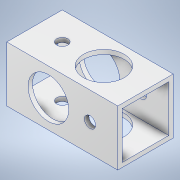
# Autodesk Inventor part: ロボットベース15x15x30
Saved by Autodesk Inventor 2020.3 (Build 243373000, 373)
## iProperties
Created: 2020-07-04
Part Number: ロボットベース15x15x30
Material: アルミニウム 6061
Document SubType Name: Modeling
Designer: totot
Density: 2.7 g/cm^3
Appearance: アルミニウム - フラット
Mass: 4.65802 g
Surface Area: 31.3598 cm^2
Volume: 1.72519 cm^3
Author: totot
Autodesk Inventor part; units mm, degrees
ref_plane "YZ Plane" through (0, 0, 0) normal (1, 0, 0) x (0, 1, 0)
ref_plane "XZ Plane" through (0, 0, 0) normal (0, 1, 0) x (-1, 0, 0)
ref_plane "XY Plane" through (0, 0, 0) normal (0, 0, 1) x (1, 0, 0)
sketch "スケッチ1" plane through (0, 0, 0) normal (1, 0, 0) x (0, 1, 0)
  line L0 (0, 0) -> (-15, 0)
  line L1 (-15, 0) -> (-15, 15)
  line L2 (-15, 15) -> (0, 15)
  line L3 (0, 15) -> (0, 0)
  line L4 (-13.8, 1.2) -> (-1.2, 1.2)
  line L5 (-1.2, 1.2) -> (-1.2, 13.8)
  line L6 (-1.2, 13.8) -> (-13.8, 13.8)
  line L7 (-13.8, 13.8) -> (-13.8, 1.2)
  dimension "d0" = 15
  dimension "d1" = 15
  dimension "d2" = 1.2
  dimension "d3" = 1.2
  dimension "d4" = 1.2
  dimension "d5" = 1.2
  constraints: 16 end point, 4 parallel, 2 horizontal, 2 perpendicular
  measures "d0" distance of L1.end L2.end
  measures "d1" distance of L0.end L1.end
  measures "d2" distance between parallel lines of L7 L1
  measures "d3" distance between parallel lines of L4 L0
  measures "d4" distance between parallel lines of L3 L5
  measures "d5" distance between parallel lines of L2 L6
extrude "押し出し1" add sketch "スケッチ1" along normal blind 30
sketch "スケッチ2" plane through (0, -15, 15) normal (0, 0, 1) x (1, 0, 0)
  line L0 (0, 0) -> (30, 0) projected
  line L1 (30, 15) -> (30, 0) projected
  point P0 (0, 15)
  point P1 (22.5, 7.5)
  dimension "d8" = 7.5
  dimension "d9" = 7.5
  measures "d8" distance from line of point (22.5, 7.5) L0
  measures "d9" distance from line of point (22.5, 7.5) L1
sketch "スケッチ3" plane through (0, 0, 15) normal (0, 1, 0) x (1, 0, 0)
  line L0 (0, 15) -> (0, 0) projected
  line L1 (0, 15) -> (30, 15) projected
  point P0 (7.5, 7.5)
  dimension "d10" = 7.5
  dimension "d11" = 7.5
  measures "d10" distance from line of point (7.5, 7.5) L0
  measures "d11" distance from line of point (7.5, 7.5) L1
hole "穴1" at (22.5, -7.5, 15) direction (0, 0, -1) diameter 3 end through all
hole "穴2" at (7.5, 0, 7.5) direction (0, -1, 0) diameter 3 end through all
sketch "スケッチ4" plane through (0, -15, 15) normal (0, 0, 1) x (1, 0, 0)
  circle A0 centre (22.5, 7.5) radius 1.5 projected
  line L0 (0, 15) -> (0, 0) projected
  line L1 (0, 15) -> (30, 15) projected
  point P0 (11.25, 7.5)
  dimension "d26" = 22.5
  dimension "d27" = 11.25
  dimension "d28" = 7.5
  measures "d26" distance from line of A0.centre L0
  measures "d27" distance from line of point (11.25, 7.5) L0
  measures "d28" distance from line of L1 point (11.25, 7.5)
hole "穴3" at (11.25, -7.5, 15) direction (0, 0, -1) diameter 11 end through all
sketch "スケッチ5" plane through (0, 0, 15) normal (0, 1, 0) x (1, 0, 0)
  line L0 (30, 15) -> (30, 0) projected
  circle A0 centre (7.5, 7.5) radius 1.5 projected
  line L1 (0, 15) -> (30, 15) projected
  point P0 (18.75, 7.5)
  dimension "d36" = 22.5
  dimension "d37" = 11.25
  dimension "d38" = 7.5
  measures "d36" distance from line of L0 A0.centre
  measures "d37" distance of point (18.75, 7.5) A0.centre
  measures "d38" distance from line of point (18.75, 7.5) L1
hole "穴4" at (18.75, 0, 7.5) direction (0, -1, 0) diameter 11 end through all
equation "\"d3\" = d2"
equation "\"d4\" = d3"
equation "\"d5\" = d4"
equation "\"d9\" = d8"
equation "\"d11\" = d10"
equation "\"d27\" = 0.5 * d26"
equation "\"d37\" = 0.5 * d36"
